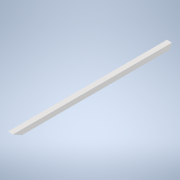
# Autodesk Inventor part: hypotAluminumExtrusion
Saved by Autodesk Inventor 2020.2 (Build 242310000, 310)
## iProperties
Created: 2020-01-19
Part Number: hypotAluminumExtrusion
Material: Generic
Document SubType Name: Modeling
Designer: robst
Density: 1 g/cm^3
Appearance: Default
Author: robst
Autodesk Inventor part; units mm, degrees
ref_plane "YZ Plane" through (0, 0, 0) normal (1, 0, 0) x (0, 1, 0)
ref_plane "XZ Plane" through (0, 0, 0) normal (0, 1, 0) x (-1, 0, 0)
ref_plane "XY Plane" through (0, 0, 0) normal (0, 0, 1) x (1, 0, 0)
sketch "Sketch1" plane through (0, 0, 0) normal (0, 0, 1) x (1, 0, 0)
  line L0 (-12.7, -12.7) -> (12.7, -12.7)
  line L1 (12.7, -12.7) -> (12.7, 12.7)
  line L2 (12.7, 12.7) -> (-12.7, 12.7)
  line L3 (-12.7, 12.7) -> (-12.7, -12.7)
  line L4 (-12.7, -12.7) -> (12.7, 12.7) construction
  line L5 (12.7, -12.7) -> (-12.7, 12.7) construction
  line L6 (-9.525, -9.525) -> (9.525, -9.525)
  line L7 (9.525, -9.525) -> (9.525, 9.525)
  line L8 (9.525, 9.525) -> (-9.525, 9.525)
  line L9 (-9.525, 9.525) -> (-9.525, -9.525)
  line L10 (-9.525, -9.525) -> (9.525, 9.525) construction
  line L11 (9.525, -9.525) -> (-9.525, 9.525) construction
  point P0 (0, 0)
  dimension "d0" = 25.4
  dimension "d1" = 25.4
  dimension "d2" = 3.175
  constraints: 24 end point, 5 parallel, 4 midpoint, 3 perpendicular, 1 horizontal
  measures "d0" distance of L0.start L0.end
  measures "d1" distance of L1.end L0.end
  measures "d2" distance between parallel lines of L6 L0
extrude "Extrusion1" add sketch "Sketch1" along normal blind 736.6
sketch "Sketch2" plane through (12.7, -12.7, 0) normal (1, 0, 0) x (0, 0, -1)
  line L0 (0, 0) -> (0, 25.4) projected
  line L1 (0, 25.4) -> (-14.6647, 0)
  line L2 (0, 0) -> (-736.6, 0) projected
  line L3 (0, 0) -> (0, 25.4)
  line L4 (-14.6647, 0) -> (0, 0)
  point P0 (0, 12.7)
  dimension "d10" = 60
  constraints: 6 end point, 1 perpendicular, 1 point on line, 1 vertical
  measures "d10" angle of L1 L2
extrude "Extrusion2" cut sketch "Sketch2" against normal through all
sketch "Sketch3" plane through (12.7, -12.7, 736.6) normal (1, 0, 0) x (0, 0, -1)
  line L0 (736.6, 25.4) -> (0, 25.4) projected
  line L1 (0, 25.4) -> (43.9941, 0)
  line L2 (721.9353, 0) -> (0, 0) projected
  line L3 (0, 0) -> (0, 25.4)
  line L4 (0, 3.175) -> (0, 22.225) projected
  line L5 (43.9941, 0) -> (0, 0)
  point P0 (736.6, 12.7)
  dimension "d7" = 30
  constraints: 6 end point, 1 collinear, 1 perpendicular, 1 point on line
  measures "d7" angle of L1 L2
extrude "Extrusion3" cut sketch "Sketch3" against normal through all
body "Solid1"
